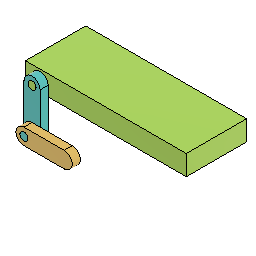
teste v1 (Autodesk Fusion 360 design; units mm, degrees)
Autodesk Fusion 360 part; units mm, degrees
note: some values were not read from the file. Set by a fixed rule: which sketch regions a step uses.
sketch "Sketch1" plane through (0, 0, 0) normal (0, 1, 0) x (1, 0, 0) in component "QUADRIL"
  line L0 (0, 0) -> (200, 0)
  line L1 (200, 0) -> (200, -25)
  line L2 (200, -25) -> (0, -25)
  line L3 (0, -25) -> (0, 0)
  dimension "d1" = 200
  dimension "d2" = 25
  constraint horizontal L0
  constraint vertical L1
  constraint horizontal L2
  constraint vertical L3
  constraint coincident L0.start L3.end
  measures "d1" distance of L0.start L0.end
  measures "d2" distance of L0.start L2.end
extrude "Extrude1" add sketch "Sketch1" along normal blind 75 makes body 1 in component "QUADRIL"
sketch "Sketch2" plane through (0, 0, 0) normal (0, -1, 0) x (1, 0, 0) in component "QUADRIL"
  line L0 (200, 25) -> (0, 25)
  line L1 (0, 25) -> (0, 0)
  line L2 (0, 0) -> (200, 0)
  line L3 (200, 0) -> (200, 25)
  circle A0 centre (18.1054, 12.5) radius 5
  dimension "d5" = 10
  dimension "d6" = 12.5
  dimension "d7" = 18.1054
  measures "d5" diameter of A0
  measures "d6" vertical distance of L1.end A0.centre
  measures "d7" horizontal distance of L1.end A0.centre
extrude "Extrude2" add sketch "Sketch2" along normal blind 10 contours A0 bodies 1 in component "QUADRIL"
sketch "Sketch2 (2)" plane through (0, 0, 0) normal (0, 1, 0) x (1, 0, 0) in component "COXA"
  circle A0 centre (18.1054, -12.5) radius 5
  circle A1 centre (18.1054, -12.5) radius 10
  line L0 (8.1054, -12.5) -> (28.1054, -12.5)
  line L1 (28.1054, -12.5) -> (28.1054, 37.5)
  line L2 (28.1054, 37.5) -> (8.1054, 37.5)
  line L3 (8.1054, 37.5) -> (8.1054, -12.5)
  circle A2 centre (18.1054, 37.5) radius 10
  circle A3 centre (18.1054, 37.5) radius 5
  dimension "d10" = 20
  dimension "d11" = 50
  dimension "d14" = 10
  constraint concentric A0 A1
  constraint perpendicular L0 L1
  constraint parallel L0 L2
  constraint parallel L1 L3
  constraint coincident A1 L0.end
  constraint horizontal L0
  constraint coincident A1 L0.start
  constraint midpoint L2 A2.centre
  constraint coincident L1.end A2
  constraint concentric A2 A3
  measures "d10" diameter of A1
  measures "d11" distance of L0.start L2.end
  measures "d14" diameter of A3
extrude "Extrude1'" add sketch "Sketch2 (2)" against normal blind 10 separate body contours A0 A1 L0 | A0 A1 L0 | A1 L1 L3 A2 | L2 A2 A3 | L2 A2 A3 makes body 2 in component "COXA"
sketch "Sketch1 (2)" plane through (0, -10, 0) normal (0, -1, 0) x (1, 0, 0) in component "PERNA"
  circle A0 centre (18.1054, 12.5) radius 5
  circle A1 centre (18.1054, -37.5) radius 5
  arc A2 (8.1054, -37.5) -> (28.1054, -37.5) centre (18.1054, -37.5) ccw
  line L0 (28.1054, -37.5) -> (28.1054, 12.5)
  arc A3 (28.1054, 12.5) -> (8.1054, 12.5) centre (18.1054, 12.5) ccw
  line L1 (8.1054, 12.5) -> (8.1054, -37.5)
  circle A4 centre (18.1054, -37.5) radius 5
  circle A5 centre (18.1054, -37.5) radius 10
  line L2 (18.1054, -47.5) -> (18.1054, -27.5)
  line L3 (18.1054, -27.5) -> (68.1054, -27.5)
  line L4 (68.1054, -27.5) -> (68.1054, -47.5)
  line L5 (68.1054, -47.5) -> (18.1054, -47.5)
  circle A6 centre (68.1054, -37.5) radius 10
  dimension "d15" = 50
  constraint concentric A4 A5
  constraint perpendicular L2 L3
  constraint parallel L2 L4
  constraint parallel L3 L5
  constraint coincident A5 L2.end
  constraint vertical L2
  constraint midpoint A2 L2.start
  constraint midpoint L4 A6.centre
  constraint coincident L4.end A6
  measures "d15" distance of L2.start L4.end
extrude "Extrude1''" add sketch "Sketch1 (2)" along normal blind 10 separate body contours A1 A2 A4 A5 L2 | A1 A2 A4 A5 L2 | L0 A5 L3 | A2 L0 A5 L3 L5 A6 | L4 A6 | L4 A6 makes body 3 in component "PERNA"
sketch "Sketch3" plane through (0, -10, 0) normal (0, -1, 0) x (1, 0, 0) in component "COXA"
  circle A0 centre (18.1054, 12.5) radius 5
  circle A1 centre (18.1054, -37.5) radius 5
  arc A2 (8.1054, -37.5) -> (28.1054, -37.5) centre (18.1054, -37.5) ccw
  line L0 (28.1054, -37.5) -> (28.1054, 12.5)
  arc A3 (28.1054, 12.5) -> (8.1054, 12.5) centre (18.1054, 12.5) ccw
  line L1 (8.1054, 12.5) -> (8.1054, -37.5)
  circle A4 centre (18.1054, -37.5) radius 5
extrude "Extrude2'" add sketch "Sketch3" along normal blind 10 and the other way blind 10 draft 10 separate body contours A1 A4 makes body 4 in component "COXA"
component "PERNA" placed x (1, 0, 0) y (0, 1, 0) z (0, 0, 1) at (0, 0, 0)
component "COXA" placed x (1, 0, 0) y (0, 1, 0) z (0, 0, 1) at (0, 0, 0)
component "QUADRIL" placed x (1, 0, 0) y (0, 1, 0) z (0, 0, 1) at (0, 0, 0)
